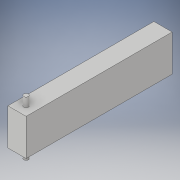
# Autodesk Inventor part: StressArm
Saved by Autodesk Inventor 2017 (Build 210142000, 142)
## iProperties
Created: 2018-03-23
Part Number: StressArm
Material: Generic
Document SubType Name: Modeling
Designer: User
Density: 1 g/cm^3
Appearance: Default
Mass: 262.997 g
Surface Area: 340.55 cm^2
Volume: 262.997 cm^3
Author: User
Autodesk Inventor part; units mm, degrees
ref_plane "YZ Plane" through (0, 0, 0) normal (1, 0, 0) x (0, 1, 0)
ref_plane "XZ Plane" through (0, 0, 0) normal (0, 1, 0) x (-1, 0, 0)
ref_plane "XY Plane" through (0, 0, 0) normal (0, 0, 1) x (1, 0, 0)
sketch "Sketch1" plane through (0, 0, 0) normal (1, 0, 0) x (0, 1, 0)
  line L0 (0, 0) -> (50.8, 0)
  line L1 (50.8, 0) -> (50.8, -203.2)
  line L2 (50.8, -203.2) -> (0, -203.2)
  line L3 (0, -203.2) -> (0, 0)
  dimension "d0" = 50.8
  dimension "d1" = 203.2
  constraints: 8 end point, 2 parallel, 1 horizontal, 1 perpendicular
  measures "d0" distance of L1.end L2.end
  measures "d1" distance of L0.end L1.end
extrude "Extrusion1" add sketch "Sketch1" along normal blind 25.4
sketch "Sketch2" plane through (0, 50.8, 0) normal (0, 1, 0) x (1, 0, 0)
  circle A0 centre (12.7, 12.7) radius 3.175
  line L0 (0, 0) -> (0, 203.2) projected
  line L1 (0, 0) -> (25.4, 0) projected
  line L2 (25.4, 203.2) -> (25.4, 0) projected
  line L3 (0, 203.2) -> (25.4, 203.2) projected
  point P0 (0, 0)
  dimension "d4" = 6.35
  dimension "d5" = 12.7
  dimension "d6" = 12.7
  constraints: 1 centre point
  measures "d4" diameter of A0
  measures "d5" distance from line of L0 A0.centre
  measures "d6" distance from line of L1 A0.centre
extrude "Extrusion2" add sketch "Sketch2" along normal blind 12.7 contours A0
sketch "Sketch3" plane through (0, 0, -203.2) normal (0, -1, 0) x (1, 0, 0)
  line L0 (0, 0) -> (0, 203.2) projected
  line L1 (0, 0) -> (25.4, 0) projected
  line L2 (25.4, 203.2) -> (25.4, 0) projected
  line L3 (0, 203.2) -> (25.4, 203.2) projected
  circle A0 centre (12.7, 190.5) radius 3.175
  dimension "d9" = 6.35
  dimension "d10" = 12.7
  dimension "d11" = 12.7
  constraints: 1 centre point
  measures "d9" diameter of A0
  measures "d10" distance from line of L2 A0.centre
  measures "d11" distance from line of L3 A0.centre
extrude "Extrusion3" add sketch "Sketch3" along normal blind 12.7 contours A0
body "Solid1"
